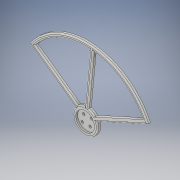
# Autodesk Inventor part: guard_F330_right
Saved by Autodesk Inventor 2019 (Build 230136000, 136)
## iProperties
Created: 2019-10-14
Part Number: guard_F330_right
Material: 一般
Document SubType Name: Modeling
Designer: dora
Density: 1 g/cm^3
Appearance: 既定
Author: dora
Autodesk Inventor part; units mm, degrees
ref_plane "YZ Plane" through (0, 0, 0) normal (1, 0, 0) x (0, 1, 0)
ref_plane "XZ Plane" through (0, 0, 0) normal (0, 1, 0) x (-1, 0, 0)
ref_plane "XY Plane" through (0, 0, 0) normal (0, 0, 1) x (1, 0, 0)
sketch "スケッチ1" plane through (0, 0, 0) normal (0, 0, 1) x (1, 0, 0)
  arc A0 (-16.2747, 11.6248) -> (18.2047, 8.2819) centre (0, 0) ccw
  arc A1 (100.1257, 45.5504) -> (-89.5107, 63.9362) centre (0, 0) ccw
  line L0 (18.2047, 8.2819) -> (100.1257, 45.5504) construction
  line L1 (-16.2747, 11.6248) -> (-89.5107, 63.9362) construction
  line L2 (-89.5107, 63.9362) -> (-16.2747, 11.6248)
  line L3 (18.2047, 8.2819) -> (100.1257, 45.5504)
  dimension "d0" = 40
  dimension "d1" = 120
  dimension "d2" = 110
  constraints: 8 end point, 4 point on circle, 2 centre point, 2 coincident, 2 collinear
  measures "d0" diameter of A0
  measures "d1" angle of L0 L1
  measures "d2" distance of A1.centre L1.end
extrude "押し出し1" add sketch "スケッチ1" along normal blind 5
sketch "スケッチ2" plane through (0, 0, 5) normal (0, 0, 1) x (1, 0, 0)
  arc A0 (100.1257, 45.5504) -> (-89.5107, 63.9362) centre (0, 0) ccw projected
  line L0 (-89.5107, 63.9362) -> (-16.2747, 11.6248) projected
  arc A1 (-16.2747, 11.6248) -> (18.2047, 8.2819) centre (0, 0) ccw projected
  line L1 (18.2047, 8.2819) -> (100.1257, 45.5504) projected
  line L2 (92.0221, 48.4555) -> (15.206, 13.5094)
  line L3 (-12.3276, 16.1789) -> (-80.9999, 65.2305)
  line L4 (-89.5107, 63.9362) -> (-16.2747, 11.6248) projected
  line L5 (18.2047, 8.2819) -> (100.1257, 45.5504) projected
  line L6 (7.0459, 103.7611) -> (-1.0446, 20.3134)
  line L7 (13.0179, 103.1821) -> (4.9274, 19.7344)
  arc A2 (92.0221, 48.4555) -> (13.0179, 103.1821) centre (0, 0) ccw
  arc A3 (7.0459, 103.7611) -> (-80.9999, 65.2305) centre (0, 0) ccw
  arc A4 (15.206, 13.5094) -> (4.9274, 19.7344) centre (0, 0) ccw
  arc A5 (-1.0446, 20.3134) -> (-12.3276, 16.1789) centre (0, 0) ccw
  dimension "d6" = 6
  dimension "d9" = 6
  constraints: 8 end point, 8 point on circle, 4 centre point, 2 parallel, 1 coincident
  measures "d6" distance between parallel lines of L0 L3
  measures "d9" distance between parallel lines of L1 L2
extrude "押し出し2" cut sketch "スケッチ2" against normal blind 8 contours L2 A4 L7 A2 | L3 A3 L6 A5
sketch "スケッチ4" plane through (0, 0, 5) normal (0, 0, 1) x (1, 0, 0)
  arc A0 (92.0221, 48.4555) -> (13.0179, 103.1821) centre (0, 0) ccw projected
  line L0 (92.0221, 48.4555) -> (15.206, 13.5094) projected
  arc A1 (15.206, 13.5094) -> (4.9274, 19.7344) centre (0, 0) ccw projected
  line L1 (4.9274, 19.7344) -> (13.0179, 103.1821) projected
  arc A2 (-1.0446, 20.3134) -> (-12.3276, 16.1789) centre (0, 0) ccw projected
  line L2 (-12.3276, 16.1789) -> (-80.9999, 65.2305) projected
  arc A3 (7.0459, 103.7611) -> (-80.9999, 65.2305) centre (0, 0) ccw projected
  line L3 (7.0459, 103.7611) -> (-1.0446, 20.3134) projected
  arc A4 (100.1257, 45.5504) -> (-89.5107, 63.9362) centre (0, 0) ccw projected
  line L4 (-89.5107, 63.9362) -> (-16.2747, 11.6248) projected
  arc A5 (-16.2747, 11.6248) -> (18.2047, 8.2819) centre (0, 0) ccw projected
  line L5 (18.2047, 8.2819) -> (100.1257, 45.5504) projected
  circle A6 centre (0, 0) radius 15
  dimension "d15" = 30
  constraints: 1 centre point, 1 coincident
  measures "d15" diameter of A6
extrude "押し出し3" cut sketch "スケッチ4" against normal blind 3 contours A6
sketch "スケッチ5" plane through (0, 0, 0) normal (0, 0, -1) x (-1, 0, 0)
  arc A0 (-13.0179, 103.1821) -> (-92.0221, 48.4555) centre (0, 0) ccw projected
  line L0 (-13.0179, 103.1821) -> (-4.9274, 19.7344) projected
  arc A1 (-4.9274, 19.7344) -> (-15.206, 13.5094) centre (0, 0) ccw projected
  line L1 (-15.206, 13.5094) -> (-92.0221, 48.4555) projected
  arc A2 (12.3276, 16.1789) -> (1.0446, 20.3134) centre (0, 0) ccw projected
  line L2 (1.0446, 20.3134) -> (-7.0459, 103.7611) projected
  arc A3 (80.9999, 65.2305) -> (-7.0459, 103.7611) centre (0, 0) ccw projected
  line L3 (80.9999, 65.2305) -> (12.3276, 16.1789) projected
  arc A4 (89.5107, 63.9362) -> (-100.1257, 45.5504) centre (0, 0) ccw projected
  line L4 (-18.2047, 8.2819) -> (-100.1257, 45.5504) projected
  arc A5 (-18.2047, 8.2819) -> (16.2747, 11.6248) centre (0, 0) ccw projected
  line L5 (89.5107, 63.9362) -> (16.2747, 11.6248) projected
  arc A6 (88.112, 64.166) -> (-98.7972, 46.0447) centre (0, 0) ccw
  line L6 (88.112, 64.166) -> (14.8583, 11.842)
  line L7 (-16.8564, 8.7671) -> (-98.7972, 46.0447)
  arc A7 (-12.1214, 104.298) -> (-93.3957, 47.9818) centre (0, 0) ccw
  line L8 (-12.1214, 104.298) -> (-3.847, 18.9538)
  line L9 (-14.9352, 12.2876) -> (-93.3957, 47.9818)
  line L10 (0.1343, 19.3398) -> (-8.14, 104.684)
  arc A8 (82.4389, 65.0294) -> (-8.14, 104.684) centre (0, 0) ccw
  line L11 (82.4389, 65.0294) -> (12.2966, 14.9278)
  line L12 (-3.847, 18.9538) -> (0.1343, 19.3398)
  line L13 (12.2966, 14.9278) -> (14.8583, 11.842)
  line L14 (-14.9352, 12.2876) -> (-16.8564, 8.7671)
  dimension "d18" = 1
  dimension "d19" = 1
  dimension "d20" = 1
  constraints: 18 end point, 6 point on circle, 3 centre point, 4 other
  measures "d18" distance between parallel lines of L7 L4
  measures "d19" distance between parallel lines of L1 L9
  measures "d20" distance between parallel lines of L11 L3
extrude "押し出し4" cut sketch "スケッチ5" against normal blind 4 contours L6 L13 L11 A8 L10 L12 L8 A7 L9 L14 L7 A6
sketch "スケッチ7" plane through (0, 0, 2) normal (0, 0, 1) x (1, 0, 0)
  circle A0 centre (0, 0) radius 15 projected
  arc A1 (92.0221, 48.4555) -> (13.0179, 103.1821) centre (0, 0) ccw projected
  line L0 (92.0221, 48.4555) -> (15.206, 13.5094) projected
  arc A2 (15.206, 13.5094) -> (4.9274, 19.7344) centre (0, 0) ccw projected
  line L1 (4.9274, 19.7344) -> (13.0179, 103.1821) projected
  arc A3 (-1.0446, 20.3134) -> (-12.3276, 16.1789) centre (0, 0) ccw projected
  line L2 (-12.3276, 16.1789) -> (-80.9999, 65.2305) projected
  arc A4 (7.0459, 103.7611) -> (-80.9999, 65.2305) centre (0, 0) ccw projected
  line L3 (7.0459, 103.7611) -> (-1.0446, 20.3134) projected
  arc A5 (100.1257, 45.5504) -> (-89.5107, 63.9362) centre (0, 0) ccw projected
  line L4 (-89.5107, 63.9362) -> (-16.2747, 11.6248) projected
  arc A6 (-16.2747, 11.6248) -> (18.2047, 8.2819) centre (0, 0) ccw projected
  line L5 (18.2047, 8.2819) -> (100.1257, 45.5504) projected
  circle A7 centre (-7.3344, -6.0379) radius 2
  circle A8 centre (-5.0846, 6.1763) radius 2
  circle A9 centre (5.0846, -6.1763) radius 2
  circle A10 centre (7.3344, 6.0379) radius 2
  circle A11 centre (0, 0) radius 15 projected
  arc A12 (92.0221, 48.4555) -> (13.0179, 103.1821) centre (0, 0) ccw projected
  line L6 (92.0221, 48.4555) -> (15.206, 13.5094) projected
  arc A13 (15.206, 13.5094) -> (4.9274, 19.7344) centre (0, 0) ccw projected
  line L7 (4.9274, 19.7344) -> (13.0179, 103.1821) projected
  arc A14 (-1.0446, 20.3134) -> (-12.3276, 16.1789) centre (0, 0) ccw projected
  line L8 (-12.3276, 16.1789) -> (-80.9999, 65.2305) projected
  arc A15 (7.0459, 103.7611) -> (-80.9999, 65.2305) centre (0, 0) ccw projected
  line L9 (7.0459, 103.7611) -> (-1.0446, 20.3134) projected
  arc A16 (100.1257, 45.5504) -> (-89.5107, 63.9362) centre (0, 0) ccw projected
  line L10 (-89.5107, 63.9362) -> (-16.2747, 11.6248) projected
  arc A17 (-16.2747, 11.6248) -> (18.2047, 8.2819) centre (0, 0) ccw projected
  line L11 (18.2047, 8.2819) -> (100.1257, 45.5504) projected
  arc A18 (100.1257, 45.5504) -> (-89.5107, 63.9362) centre (0, 0) ccw projected
  line L12 (7.0459, 103.7611) -> (-1.0446, 20.3134) projected
  line L13 (10.3271, 106.5166) -> (10.036, 103.5146)
  line L14 (1.9628, 20.2453) -> (1.8563, 19.1468)
  line L15 (10.615, 109.4866) -> (10.5185, 108.4913)
  dimension "d23" = 4
  dimension "d25" = 4
  dimension "d26" = 4
  dimension "d27" = 16
  dimension "d29" = 4
  dimension "d30" = 19
  constraints: 6 end point, 4 centre point, 4 point on circle, 1 parallel
  measures "d23" diameter of A7
  measures "d25" diameter of A8
  measures "d26" diameter of A9
  measures "d27" distance of A9.centre A8.centre
  measures "d29" diameter of A10
  measures "d30" distance of A10.centre A7.centre
extrude "押し出し5" cut sketch "スケッチ7" against normal blind 10 contours A7 | A8 | A9 | A10
fillet "フィレット1" radius 2 8 edges at (10.615, 109.4866, 5) (59.1652, 26.9162, 5) (8.9726, 61.4582, 5) (3.0006, 62.0372, 5) (-46.6637, 40.7047, 5) (-52.8927, 37.7805, 5) (-41.6947, 95.2762, 5) (59.2207, 85.4921, 5)
fillet "フィレット2" radius 2 3 edges at (10.5369, 17.3983, 5) (-6.9984, 19.0984, 5) (-1.93, -19.9067, 5)
